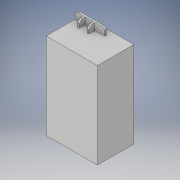
# Autodesk Inventor part: Battery
Saved by Autodesk Inventor 2019.3 (Build 233278000, 278)
## iProperties
Created: 2019-01-26
Part Number: Battery
Material: Generic
Document SubType Name: Modeling
Designer: mark
Density: 1 g/cm^3
Appearance: Default
Author: mark
Autodesk Inventor part; units mm, degrees
ref_plane "YZ Plane" through (0, 0, 0) normal (1, 0, 0) x (0, 1, 0)
ref_plane "XZ Plane" through (0, 0, 0) normal (0, 1, 0) x (-1, 0, 0)
ref_plane "XY Plane" through (0, 0, 0) normal (0, 0, 1) x (1, 0, 0)
sketch "Sketch1" plane through (0, 0, 0) normal (0, 0, 1) x (1, 0, 0)
  line L0 (0, 0) -> (83, 0)
  line L1 (83, 0) -> (83, 139.7)
  line L2 (83, 139.7) -> (0, 139.7)
  line L3 (0, 139.7) -> (0, 0)
  dimension "d0" = 83
  dimension "d1" = 139.7
  constraints: 8 end point
  measures "d0" distance of L2.end L1.end
  measures "d1" distance of L1.end L0.end
extrude "Extrusion1" add sketch "Sketch1" along normal blind 59.1
sketch "Sketch2" plane through (0, 139.7, 0) normal (0, 1, 0) x (1, 0, 0)
  line L0 (0, -9) -> (47.7, -9)
  line L1 (47.7, -9) -> (47.7, -12)
  line L2 (47.7, -12) -> (0, -12)
  line L3 (0, -12) -> (0, -9)
  line L4 (83, 0) -> (0, 0) projected
  line L5 (13, -12) -> (16, -12)
  line L6 (16, -12) -> (16, -21.7)
  line L7 (16, -21.7) -> (13, -21.7)
  line L8 (13, -21.7) -> (13, -12)
  line L9 (0, 0) -> (0, -59.1) projected
  line L10 (29, -12) -> (32, -12)
  line L11 (32, -12) -> (32, -21.7)
  line L12 (32, -21.7) -> (29, -21.7)
  line L13 (29, -21.7) -> (29, -12)
  dimension "d4" = 3
  dimension "d5" = 47.7
  dimension "d6" = 9
  dimension "d7" = 9.7
  dimension "d8" = 3
  dimension "d9" = 13
  dimension "d10" = 3
  dimension "d11" = 9.7
  dimension "d12" = 29
  constraints: 24 end point, 3 point on line, 2 perpendicular
  measures "d4" distance between parallel lines of L0 L2
  measures "d5" distance between parallel lines of L1 L3
  measures "d6" distance between parallel lines of L0 L4
  measures "d7" distance between parallel lines of L2 L7
  measures "d8" distance between parallel lines of L8 L6
  measures "d9" distance between parallel lines of L9 L8
  measures "d10" distance between parallel lines of L11 L13
  measures "d11" distance between parallel lines of L12 L10
  measures "d12" distance between parallel lines of L9 L13
extrude "Extrusion2" add sketch "Sketch2" along normal blind 11.37
sketch "Sketch3" plane through (0, 0, 0) normal (0, -1, 0) x (1, 0, 0)
  line L0 (83, 0) -> (0, 0)
  line L1 (0, 9) -> (47.7, 9)
  line L2 (47.7, 9) -> (47.7, 12)
  line L3 (47.7, 12) -> (0, 12)
  line L4 (0, 12) -> (0, 9)
  line L5 (13, 12) -> (16, 12)
  line L6 (16, 12) -> (16, 21.7)
  line L7 (16, 21.7) -> (13, 21.7)
  line L8 (13, 21.7) -> (13, 12)
  line L9 (0, 0) -> (0, 59.1)
  line L10 (29, 12) -> (32, 12)
  line L11 (32, 12) -> (32, 21.7)
  line L12 (32, 21.7) -> (29, 21.7)
  line L13 (29, 21.7) -> (29, 12)
  constraints: 28 end point, 3 point on line
extrude "Extrusion3" add sketch "Sketch3" along normal blind 11.37
fillet "Fillet1" radius 5 4 edges at (0, 151.07, 10.5) (47.7, 151.07, 10.5) (0, -11.37, 10.5) (47.7, -11.37, 10.5)
chamfer "Chamfer1" distance 5 angle 45 4 edges at (30.5, -11.37, 21.7) (14.5, -11.37, 21.7) (30.5, 151.07, 21.7) (14.5, 151.07, 21.7)
body "Solid1"
